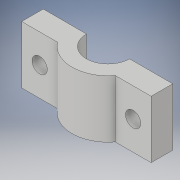
# Autodesk Inventor part: innerCrutchAttacement
Saved by Autodesk Inventor 2017 SP1 (Build 210196100, 196)
## iProperties
Created: 2016-07-31
Part Number: innerCrutchAttacement
Material: Generic
Document SubType Name: Modeling
Designer: steele
Density: 1 g/cm^3
Appearance: Default
Author: steele
Autodesk Inventor part; units mm, degrees
ref_plane "YZ Plane" through (0, 0, 0) normal (1, 0, 0) x (0, 1, 0)
ref_plane "XZ Plane" through (0, 0, 0) normal (0, 1, 0) x (-1, 0, 0)
ref_plane "XY Plane" through (0, 0, 0) normal (0, 0, 1) x (1, 0, 0)
sketch "Sketch1" plane through (0, 0, 0) normal (0, 1, 0) x (-1, 0, 0)
  line L0 (0, 0) -> (0, 38.1) construction
  line L1 (0, 0) -> (0, -38.1) construction
  arc A0 (-9.525, -38.1) -> (9.525, -38.1) centre (0, -38.1) ccw construction
  circle A1 centre (0, 38.1) radius 9.525 construction
  line L2 (15.875, -38.1) -> (28.575, -38.1)
  line L3 (15.875, -38.1) -> (-15.875, -38.1) construction
  line L4 (15.875, -38.1) -> (9.525, -38.1)
  line L5 (-9.525, -38.1) -> (-15.875, -38.1)
  arc A2 (9.525, -38.1) -> (-9.525, -38.1) centre (0, -38.1) ccw construction
  arc A3 (12.7, -28.575) -> (-12.7, -28.575) centre (0, -38.1) ccw
  arc A4 (9.525, -38.1) -> (-9.525, -38.1) centre (0, -38.1) ccw
  line L6 (28.575, -38.1) -> (28.575, -28.575)
  line L7 (28.575, -28.575) -> (12.7, -28.575)
  line L8 (-15.875, -38.1) -> (-28.575, -38.1)
  line L9 (-28.575, -38.1) -> (-28.575, -28.575)
  line L10 (-28.575, -28.575) -> (-12.7, -28.575)
  point P0 (-101.6, -47.625)
  dimension "d0" = 76.2
  dimension "d1" = 19.05
  dimension "d9" = 9.525
  dimension "d17" = 15.875
  dimension "d18" = 15.875
  constraints: 22 end point, 8 point on circle, 5 centre point, 4 coincident, 4 collinear, 3 horizontal, 3 vertical, 2 perpendicular, 2 point on line, 1 equal radius, 1 parallel
  measures "d0" distance of L0.end L1.end
  measures "d1" diameter of A0
  measures "d9" distance of L2.end L6.end
  measures "d17" distance of L6.end L7.end
  measures "d18" distance of L9.end L10.end
extrude "Extrusion1" add sketch "Sketch1" along normal mid plane 25.4
sketch "Sketch2" plane through (-28.575, 12.7, -28.575) normal (0, 0, 1) x (1, 0, 0)
  line L0 (19.05, 0) -> (0, 0) construction
  line L1 (15.875, -25.4) -> (15.875, 0) construction
  line L2 (0, 0) -> (15.875, -25.4) construction
  line L3 (15.875, -25.4) -> (0, -25.4) construction
  line L4 (15.875, 0) -> (0, -25.4) construction
  point P0 (28.575, -12.7)
  point P1 (7.9375, -12.7)
  constraints: 4 end point, 1 midpoint
hole "Hole1" at (-20.6375, 0, -28.575) direction (0, 0, -1) diameter 6.7564 end through all clearance for "Flat Head Machine Screw (82)" size "1/4" standard "Ansi Unified Screw Threads"
sketch "Sketch3" plane through (12.7, 12.7, -28.575) normal (0, 0, 1) x (1, 0, 0)
  line L0 (0, -25.4) -> (0, 0) construction
  line L1 (15.875, -25.4) -> (15.875, 0) construction
  line L2 (0, 0) -> (15.875, -25.4) construction
  line L3 (15.875, -25.4) -> (15.875, 0) construction
  line L4 (15.875, 0) -> (0, -25.4) construction
  point P0 (-12.7, -12.7)
  point P1 (7.9375, -12.7)
  constraints: 6 end point, 1 collinear, 1 midpoint
hole "Hole2" at (20.6375, 0, -28.575) direction (0, 0, -1) diameter 6.7564 end through all clearance for "Flat Head Machine Screw (82)" size "1/4" standard "Ansi Unified Screw Threads"
equation "\"d0\" = crutchTubSpacing"
equation "\"d1\" = cruchTubeDiam"
equation "\"cruchTubeDiam\" = 19.05"
equation "\"wallThickness\" = 6.35"
equation "\"crutchTubSpacing\" = 76.2"
equation "\"supportHeight\" = 25.4"
body "Solid1"
